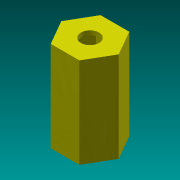
# Autodesk Inventor part: AntiBacklash
Saved by Autodesk Inventor 2016 (Build 200138000, 138)
## iProperties
Created: 2015-06-03
Part Number: AntiBacklash
Material: ABS Plastic
Document SubType Name: Modeling
Designer: Sawaiz Syed
Density: 1.06 g/cm^3
Appearance: Smooth - Yellow
Author: Sawaiz Syed
Autodesk Inventor part; units mm, degrees
ref_plane "YZ Plane" through (0, 0, 0) normal (1, 0, 0) x (0, 1, 0)
ref_plane "XZ Plane" through (0, 0, 0) normal (0, 1, 0) x (-1, 0, 0)
ref_plane "XY Plane" through (0, 0, 0) normal (0, 0, 1) x (1, 0, 0)
sketch "Sketch1" plane through (0, 0, 0) normal (0, 0, 1) x (1, 0, 0)
  line L0 (5.4993, 3.175) -> (7.3323, 0)
  line L1 (0, 6.35) -> (3.6662, 6.35)
  line L2 (3.6662, 6.35) -> (5.4993, 3.175)
  line L3 (7.3323, 0) -> (5.4993, -3.175)
  line L4 (5.4993, -3.175) -> (3.6662, -6.35)
  line L5 (3.6662, -6.35) -> (0, -6.35)
  line L6 (0, -6.35) -> (-3.6662, -6.35)
  line L7 (-3.6662, -6.35) -> (-5.4993, -3.175)
  line L8 (-5.4993, -3.175) -> (-7.3323, 0)
  line L9 (-7.3323, 0) -> (-5.4993, 3.175)
  line L10 (-5.4993, 3.175) -> (-3.6662, 6.35)
  line L11 (-3.6662, 6.35) -> (0, 6.35)
  line L12 (5.6725, 3.275) -> (7.5633, 0)
  line L13 (7.5633, 0) -> (5.6725, -3.275)
  line L14 (5.6725, -3.275) -> (3.7816, -6.55)
  line L15 (3.7816, -6.55) -> (0, -6.55)
  line L16 (0, -6.55) -> (-3.7816, -6.55)
  line L17 (-3.7816, -6.55) -> (-5.6725, -3.275)
  line L18 (-5.6725, -3.275) -> (-7.5633, 0)
  line L19 (-7.5633, 0) -> (-5.6725, 3.275)
  line L20 (-5.6725, 3.275) -> (-3.7816, 6.55)
  line L21 (-3.7816, 6.55) -> (0, 6.55)
  line L22 (0, 6.55) -> (3.7816, 6.55)
  line L23 (3.7816, 6.55) -> (5.6725, 3.275)
  line L24 (10.0026, 5.775) -> (13.3368, 0)
  line L25 (13.3368, 0) -> (10.0026, -5.775)
  line L26 (10.0026, -5.775) -> (6.6684, -11.55)
  line L27 (6.6684, -11.55) -> (0, -11.55)
  line L28 (0, -11.55) -> (-6.6684, -11.55)
  line L29 (-6.6684, -11.55) -> (-10.0026, -5.775)
  line L30 (-10.0026, -5.775) -> (-13.3368, 0)
  line L31 (-13.3368, 0) -> (-10.0026, 5.775)
  line L32 (-10.0026, 5.775) -> (-6.6684, 11.55)
  line L33 (-6.6684, 11.55) -> (0, 11.55)
  line L34 (0, 11.55) -> (6.6684, 11.55)
  line L35 (6.6684, 11.55) -> (10.0026, 5.775)
  point P0 (0, 0)
  dimension "d0" = 0.2
  dimension "d1" = 5
  constraints: 72 end point, 22 other
  measures "d0" distance between parallel lines of L2 L23
  measures "d1" distance between parallel lines of L23 L35
extrude "Extrusion1" add sketch "Sketch1" against normal blind 40 contours L24 L25 L26 L27 L28 L29 L30 L31 L32 L33 L34 L35
sketch "Sketch2" plane through (0, 0, 0) normal (0, 0, 1) x (1, 0, 0)
  line L0 (-3.7816, 6.55) -> (3.7816, 6.55) projected
  line L1 (3.7816, 6.55) -> (7.5633, 0) projected
  line L2 (7.5633, 0) -> (3.7816, -6.55) projected
  line L3 (3.7816, -6.55) -> (-3.7816, -6.55) projected
  line L4 (-3.7816, -6.55) -> (-7.5633, 0) projected
  line L5 (-7.5633, 0) -> (-3.7816, 6.55) projected
  line L6 (6.6684, 11.55) -> (13.3368, 0) projected
  line L7 (-6.6684, 11.55) -> (6.6684, 11.55) projected
  line L8 (-13.3368, 0) -> (-6.6684, 11.55) projected
  line L9 (-6.6684, -11.55) -> (-13.3368, 0) projected
  line L10 (6.6684, -11.55) -> (-6.6684, -11.55) projected
  line L11 (13.3368, 0) -> (6.6684, -11.55) projected
  point P0 (0, 0)
extrude "Extrusion2" add sketch "Sketch2" along normal blind 2 contours L0 L1 L2 L3 L4 L5 | L6 L11 L10 L9 L8 L7
sketch "Sketch3" plane through (0, 0, 2) normal (0, 0, 1) x (1, 0, 0)
  point P0 (0, 0)
  point P1 (0, 0)
  constraints: 1 coincident
hole "Hole1" at (0, 0, 2) direction (0, 0, -1) diameter 8.4375 end through all
body "Solid1"
